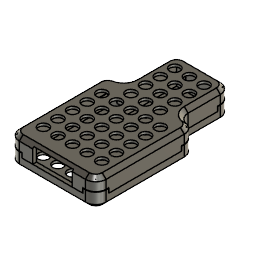
usb elrs case (Autodesk Fusion 360 design; units mm, degrees)
Autodesk Fusion 360 part; units mm, degrees
sketch "Sketch1" plane through (0, 0, 0) normal (0, 0, 1) x (1, 0, 0)
  line L0 (9.2, -10.6) -> (-9.2, -10.6)
  line L1 (-9.2, -10.6) -> (-9.2, 10.6)
  line L2 (9.2, 10.6) -> (9.2, -10.6)
  line L3 (9.2, -10.6) -> (-9.2, 10.6) construction
  line L4 (-9.2, -10.6) -> (9.2, 10.6) construction
  line L5 (0, -11.5) -> (0, 35.0108) construction
  line L6 (-5.4, 10.6) -> (-5.4, 22.8)
  line L7 (-5.4, 22.8) -> (5.4, 22.8)
  line L8 (5.4, 22.8) -> (5.4, 10.6)
  line L9 (5.4, 10.6) -> (-5.4, 22.8) construction
  line L10 (-5.4, 10.6) -> (5.4, 22.8) construction
  line L11 (-10.1, -11.5) -> (-10.1, 11.5)
  line L12 (10.1, 11.5) -> (10.1, -11.5)
  line L13 (10.1, -11.5) -> (-10.1, -11.5)
  line L14 (-6.3, 11.5) -> (-6.3, 23.7)
  line L15 (-6.3, 23.7) -> (6.3, 23.7)
  line L16 (6.3, 23.7) -> (6.3, 11.5)
  line L17 (-10.1, 11.5) -> (-6.3, 11.5)
  line L18 (6.3, 11.5) -> (10.1, 11.5)
  line L19 (-9.2, 10.6) -> (-5.4, 10.6)
  line L20 (5.4, 10.6) -> (9.2, 10.6)
  line L21 (4.6, -8.2) -> (4.6, -11.5)
  line L22 (-4.6, -11.5) -> (-4.6, -8.2)
  line L23 (-4.6, -6.5489) -> (4.6, -12.5489) construction
  line L24 (4.6, -6.5489) -> (-4.6, -12.5489) construction
  line L25 (6.8, 8.2) -> (6.8, 7.8348)
  line L26 (6.8, -7.8348) -> (6.8, -8.2)
  line L27 (-6.8, -8.2) -> (-6.8, -7.8348)
  line L28 (-6.8, 7.8348) -> (-6.8, 8.2)
  circle A0 centre (0, 0) radius 1.2
  circle A1 centre (-6.8, -6.8) radius 1.2
  circle A2 centre (-3.4, -6.8) radius 1.2
  circle A3 centre (0, -6.8) radius 1.2
  circle A4 centre (3.4, -6.8) radius 1.2
  circle A5 centre (6.8, -6.8) radius 1.2
  circle A6 centre (-6.8, -3.4) radius 1.2
  circle A7 centre (-3.4, -3.4) radius 1.2
  circle A8 centre (0, -3.4) radius 1.2
  circle A9 centre (3.4, -3.4) radius 1.2
  circle A10 centre (6.8, -3.4) radius 1.2
  circle A11 centre (-6.8, 0) radius 1.2
  circle A12 centre (-3.4, 0) radius 1.2
  circle A13 centre (3.4, 0) radius 1.2
  circle A14 centre (6.8, 0) radius 1.2
  circle A15 centre (-6.8, 3.4) radius 1.2
  circle A16 centre (-3.4, 3.4) radius 1.2
  circle A17 centre (0, 3.4) radius 1.2
  circle A18 centre (3.4, 3.4) radius 1.2
  circle A19 centre (6.8, 3.4) radius 1.2
  circle A20 centre (-6.8, 6.8) radius 1.2
  circle A21 centre (-3.4, 6.8) radius 1.2
  circle A22 centre (0, 6.8) radius 1.2
  circle A23 centre (3.4, 6.8) radius 1.2
  circle A24 centre (6.8, 6.8) radius 1.2
  circle A25 centre (-3.4, 10.2) radius 1.2
  circle A26 centre (0, 10.2) radius 1.2
  circle A27 centre (3.4, 10.2) radius 1.2
  circle A28 centre (-3.4, 13.6) radius 1.2
  circle A29 centre (0, 13.6) radius 1.2
  circle A30 centre (3.4, 13.6) radius 1.2
  circle A31 centre (-3.4, 17) radius 1.2
  circle A32 centre (0, 17) radius 1.2
  circle A33 centre (3.4, 17) radius 1.2
  circle A34 centre (-3.4, 20.4) radius 1.2
  circle A35 centre (0, 20.4) radius 1.2
  circle A36 centre (3.4, 20.4) radius 1.2
  line L29 (10.1, 11.5) -> (7.1, 11.5)
  line L30 (7.1, 11.5) -> (7.1, 8.5)
  line L31 (7.1, 8.5) -> (10.1, 8.5)
  line L32 (10.1, 8.5) -> (10.1, 11.5)
  line L33 (-10.1, 11.5) -> (-7.1, 11.5)
  line L34 (-7.1, 11.5) -> (-7.1, 8.5)
  line L35 (-7.1, 8.5) -> (-10.1, 8.5)
  line L36 (-10.1, 8.5) -> (-10.1, 11.5)
  line L37 (-10.1, -11.5) -> (-7.1, -11.5)
  line L38 (-7.1, -11.5) -> (-7.1, -8.5)
  line L39 (-7.1, -8.5) -> (-10.1, -8.5)
  line L40 (-10.1, -8.5) -> (-10.1, -11.5)
  line L41 (10.1, -11.5) -> (7.1, -11.5)
  line L42 (7.1, -11.5) -> (7.1, -8.5)
  line L43 (7.1, -8.5) -> (10.1, -8.5)
  line L44 (10.1, -8.5) -> (10.1, -11.5)
  line L45 (-6.3, 23.7) -> (-3.3, 23.7)
  line L46 (-3.3, 23.7) -> (-3.3, 20.7)
  line L47 (-3.3, 20.7) -> (-6.3, 20.7)
  line L48 (-6.3, 20.7) -> (-6.3, 23.7)
  line L49 (6.3, 23.7) -> (3.3, 23.7)
  line L50 (3.3, 23.7) -> (3.3, 20.7)
  line L51 (3.3, 20.7) -> (6.3, 20.7)
  line L52 (6.3, 20.7) -> (6.3, 23.7)
  point P0 (0, 16.7)
  point P1 (0, -9.5489)
  dimension "d1" = 18.4
  dimension "d2" = 21.2
  dimension "d3" = 10.8
  dimension "d4" = 12.2
  dimension "d8" = 9.2
  dimension "d9" = 6
  dimension "d26" = 2.4
  dimension "d29" = 3.4
  dimension "d30" = 3.4
  dimension "d32" = 3
  dimension "d33" = 3
  dimension "d34" = 3
  dimension "d35" = 3
  dimension "d36" = 3
  dimension "d37" = 3
  dimension "d38" = 3
  dimension "d39" = 3
  dimension "d40" = 3
  dimension "d41" = 3
  dimension "d42" = 3
  dimension "d43" = 3
  constraint horizontal L0
  constraint perpendicular L0 L1
  constraint parallel L0 L19
  constraint parallel L1 L2
  constraint coincident L3 A0.centre
  constraint coincident L4 A0.centre
  constraint coincident A0.centre origin
  constraint perpendicular L5 L20
  constraint parallel L6 L8
  constraint coincident L9 P0
  constraint coincident L10 P0
  constraint coincident L5 P0
  constraint collinear L17 L18
  constraint collinear L19 L20
  constraint coincident L13 L5.start
  constraint parallel L21 L22
  constraint coincident L23 P1
  constraint coincident L24 P1
  constraint coincident L5 P1
  constraint coincident L13 L21.end
  constraint coincident L13 L22.start
  constraint coincident L4 L25.end
  constraint coincident L3 L26.start
  constraint collinear L25 L26
  constraint coincident L4 L27.end
  constraint coincident L3 L28.start
  constraint collinear L27 L28
  constraint horizontal L29
  constraint vertical L30
  constraint horizontal L31
  constraint vertical L32
  constraint horizontal L33
  constraint vertical L34
  constraint horizontal L35
  constraint vertical L36
  constraint horizontal L37
  constraint vertical L38
  constraint horizontal L39
  constraint vertical L40
  constraint horizontal L41
  constraint vertical L42
  constraint horizontal L43
  constraint vertical L44
  constraint horizontal L45
  constraint vertical L46
  constraint horizontal L47
  constraint vertical L48
  constraint horizontal L49
  constraint vertical L50
  constraint horizontal L51
  constraint vertical L52
  measures "d1" distance of L1.end L2.start
  measures "d2" distance of L0.end L1.end
  measures "d3" distance of L6.end L7.end
  measures "d4" distance of L6.start L6.end
  measures "d8" distance of L23.end L24.end
  measures "d9" distance of L24.start L23.end
  measures "d26" diameter of A0
  measures "d32" distance of L12.start L29.end
  measures "d33" distance of L12.start L31.end
  measures "d34" distance of L11.end L33.end
  measures "d35" distance of L11.end L35.end
  measures "d36" distance of L11.start L37.end
  measures "d37" distance of L11.start L39.end
  measures "d38" distance of L12.end L41.end
  measures "d39" distance of L12.end L43.end
  measures "d40" distance of L14.end L45.end
  measures "d41" distance of L14.end L47.end
  measures "d42" distance of L15.end L49.end
  measures "d43" distance of L15.end L51.end
extrude "Extrude2" add sketch "Sketch1" along normal blind 0.6 contours L0 L2 L42 L43 | L0 L1 L2 L6 L7 L8 L19 L20 A34 A36 L30 L31 L34 L35 L38 L39 L42 L43 L46 L47 L50 L51 | L2 L20 L30 L31 | L0 L1 L38 L39 | L7 L8 A36 L50 L51 | L1 L19 L34 L35 | A36 L50 L51 | A36 L50 L51 | L6 L7 A34 L46 L47 | A34 L46 L47 | A34 L46 L47 | A0 | A1 | A2 | A3 | A4 | A5 | A6 | A7 | A8 | A9 | A10 | A11 | A12 | A13 | A14 | A15 | A16 | A17 | A18 | A19 | A20 | A21 | A22 | A23 | A24 | A25 | A26 | A27 | A28 | A29 | A30 | A31 | A32 | A33 | A35 makes body 1
extrude "Extrude3" add sketch "Sketch1" along normal blind 2.4 contours L0 L2 L12 L13 L41 L42 L43 L44 | L0 L13 L21 L42 | L2 L12 L31 L43 | L0 L13 L21 L22 | L2 L12 L18 L20 L29 L30 L31 L32 | L0 L13 L22 L38 | L0 L1 L11 L13 L37 L38 L39 L40 | L8 L16 L18 L20 L30 L51 | L1 L11 L35 L39 | L7 L8 L15 L16 L49 L50 L51 L52 | L1 L11 L17 L19 L33 L34 L35 L36 | L7 L15 L46 L50 | L6 L14 L17 L19 L34 L47 | L6 L7 L14 L15 L45 L46 L47 L48 bodies 1
extrude "Extrude4" add sketch "Sketch1" along normal blind 4 from surface at 2.4 separate body contours L0 L2 L12 L13 L41 L42 L43 L44 | L0 L13 L21 L42 | L2 L12 L31 L43 | L2 L12 L18 L20 L29 L30 L31 L32 | L0 L13 L22 L38 | L0 L1 L11 L13 L37 L38 L39 L40 | L8 L16 L18 L20 L30 L51 | L1 L11 L35 L39 | L7 L8 L15 L16 L49 L50 L51 L52 | L1 L11 L17 L19 L33 L34 L35 L36 | L7 L15 L46 L50 | L6 L14 L17 L19 L34 L47 | L6 L7 L14 L15 L45 L46 L47 L48 makes body 2
extrude "Extrude5" add sketch "Sketch1" against normal blind 0.6 from surface at 6.4 contours L0 L2 L42 L43 | L0 L1 L2 L6 L7 L8 L19 L20 A34 A36 L30 L31 L34 L35 L38 L39 L42 L43 L46 L47 L50 L51 | L2 L20 L30 L31 | L0 L1 L38 L39 | L7 L8 A36 L50 L51 | L1 L19 L34 L35 | A36 L50 L51 | A36 L50 L51 | L6 L7 A34 L46 L47 | A34 L46 L47 | A34 L46 L47 | A0 | A1 | A2 | A3 | A4 | A5 | A6 | A7 | A8 | A9 | A10 | A11 | A12 | A13 | A14 | A15 | A16 | A17 | A18 | A19 | A20 | A21 | A22 | A23 | A24 | A25 | A26 | A27 | A28 | A29 | A30 | A31 | A32 | A33 | A35 bodies 2
move_face "OffsetFaces1" offset 0.9 1 faces at (1.5333, -10.6, 6.2) on bodies 2
fillet "Fillet1" radius 2.4 16 edges at (10.1, -11.5, 1.2) (10.1, 11.5, 1.2) (6.3, 23.7, 1.2) (-10.1, -11.5, 1.2) (-10.1, 11.5, 1.2) (-6.3, 11.5, 1.2) (-6.3, 23.7, 1.2) (6.3, 11.5, 1.2) (10.1, -11.5, 4.4) (10.1, 11.5, 4.4) (6.3, 23.7, 4.4) (-10.1, -11.5, 4.4) (-10.1, 11.5, 4.4) (-6.3, 11.5, 4.4) (-6.3, 23.7, 4.4) (6.3, 11.5, 4.4) on bodies 1 2
chamfer "Chamfer1" distance 0.9 angle 45 28 edges at (0, -11.5, 0) (-9.3971, -10.7971, 0) (-10.1, 0, 0) (-9.5655, 10.61, 0) (-6.8345, 12.2847, 0) (-6.3, 17.5473, 0) (-5.5971, 22.9971, 0) (0, 23.7, 0) (5.5971, 22.9971, 0) (6.3, 17.5473, 0) (6.8345, 12.2847, 0) (9.5655, 10.61, 0) (10.1, 0, 0) (9.3971, -10.7971, 0) (-10.1, 0, 6.4) (-9.3971, -10.7971, 6.4) (0, -11.5, 6.4) (9.3971, -10.7971, 6.4) (10.1, 0, 6.4) (9.5655, 10.61, 6.4) (6.8345, 12.2847, 6.4) (6.3, 17.5473, 6.4) (5.5971, 22.9971, 6.4) (0, 23.7, 6.4) (-5.5971, 22.9971, 6.4) (-6.3, 17.5473, 6.4) (-6.8345, 12.2847, 6.4) (-9.5655, 10.61, 6.4) on bodies 1 2
extrude "Extrude6" cut sketch "Sketch1" along normal through all contours A36 L50 L51 | A36 L50 L51 | A34 L46 L47 | A34 L46 L47 | A0 | A1 | A2 | A3 | A4 | A5 | A6 | A7 | A8 | A9 | A10 | A11 | A12 | A13 | A14 | A15 | A16 | A17 | A18 | A19 | A20 | A21 | A22 | A23 | A24 | A25 | A26 | A27 | A28 | A29 | A30 | A31 | A32 | A33 | A35 bodies 1 2
sketch "Sketch2" plane through (0, 0, 2.4) normal (0, 0, 1) x (-1, 0, 0)
  line L0 (-5.4, -22.8) -> (-5.4, -10.6)
  line L1 (-5.4, -10.6) -> (-9.2, -10.6)
  line L2 (-9.2, -10.6) -> (-9.2, 10.6)
  line L3 (-9.2, 10.6) -> (9.2, 10.6)
  line L4 (9.2, 10.6) -> (9.2, -10.6)
  line L5 (9.2, -10.6) -> (5.4, -10.6)
  line L6 (5.4, -10.6) -> (5.4, -22.8)
  line L7 (5.4, -22.8) -> (-5.4, -22.8)
  arc A0 (3.9, -23.7) -> (6.3, -21.3) centre (3.9, -21.3) ccw
  line L8 (6.3, -21.3) -> (6.3, -13.7947)
  arc A1 (8.2, -11.4473) -> (6.3, -13.7947) centre (8.7, -13.7947) ccw
  arc A2 (8.2, -11.4473) -> (10.1, -9.1) centre (7.7, -9.1) ccw
  line L9 (10.1, -9.1) -> (10.1, 9.1)
  arc A3 (10.1, 9.1) -> (7.7, 11.5) centre (7.7, 9.1) ccw
  line L10 (7.7, 11.5) -> (-7.7, 11.5)
  arc A4 (-7.7, 11.5) -> (-10.1, 9.1) centre (-7.7, 9.1) ccw
  line L11 (-10.1, 9.1) -> (-10.1, -9.1)
  arc A5 (-10.1, -9.1) -> (-8.2, -11.4473) centre (-7.7, -9.1) ccw
  arc A6 (-6.3, -13.7947) -> (-8.2, -11.4473) centre (-8.7, -13.7947) ccw
  line L12 (-6.3, -13.7947) -> (-6.3, -21.3)
  arc A7 (-6.3, -21.3) -> (-3.9, -23.7) centre (-3.9, -21.3) ccw
  line L13 (-3.9, -23.7) -> (3.9, -23.7)
  line L14 (7.1, 11.5) -> (7.1, 8.5)
  line L15 (7.1, 8.5) -> (10.1, 8.5)
  line L16 (-7.1, 11.5) -> (-7.1, 8.5)
  line L17 (-7.1, 8.5) -> (-10.1, 8.5)
  line L18 (7.1, -8.5) -> (10.1, -8.5)
  line L19 (7.1, -11.5) -> (7.1, -8.5)
  line L20 (-7.1, -11.5) -> (-7.1, -8.5)
  line L21 (-7.1, -8.5) -> (-10.1, -8.5)
  line L22 (3.3, -23.7) -> (3.3, -20.7)
  line L23 (-3.3, -23.7) -> (-3.3, -20.7)
  line L24 (-3.3, -20.7) -> (-6.3, -20.7)
  line L25 (-7.1, -8.5) -> (-7.1, -12.4312)
  line L26 (7.1, -8.5) -> (7.1, -12.4373)
  line L27 (3.3, -20.7) -> (7.0554, -20.7)
  constraint coincident L20.end L21.start
  constraint perpendicular L21 L25
  constraint coincident L18.start L19.end
  constraint perpendicular L18 L26
  constraint coincident L22.end L27.start
  constraint perpendicular L8 L27
extrude "Extrude7" add sketch "Sketch2" along normal blind 1 contours L0 L7 L12 A7 L13 L23 L24 | L6 L7 A0 L8 L13 L22 L27 | L1 L2 L11 A5 A6 L20 L21 L25 | L2 L3 L10 A4 L11 L16 L17 | L4 L5 A1 A2 L9 L18 L19 L26 | L3 L4 L9 A3 L10 L14 L15 bodies 1
extrude "Extrude8" cut sketch "Sketch2" along normal blind 1.1 contours L0 L7 L12 A7 L13 L23 L24 | L6 L7 A0 L8 L13 L22 L27 | L1 L2 L11 A5 A6 L20 L21 L25 | L2 L3 L10 A4 L11 L16 L17 | L4 L5 A1 A2 L9 L18 L19 L26 | L3 L4 L9 A3 L10 L14 L15 bodies 2
move_face "OffsetFaces2" offset -0.05 12 faces at (9.8, 8.5, 3.1333) (-9.8, 8.5, 3.1333) (-7.1, 11.0686, 2.7667) (7.1, 11.5372, 2.7667) (6, 20.7, 3.1333) (3.3, 23.4, 2.7667) (-3.3, 23.4, 2.7667) (-5.7, 20.7, 2.7667) (9.8, -8.5, 3.1333) (7.1, -10.9, 3.1333) (-7.1, -10.9, 3.1333) (-9.8, -8.5, 3.1333) on bodies 2
